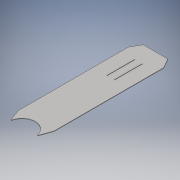
# Autodesk Inventor part: Table
Saved by Autodesk Inventor 2016 (Build 200138000, 138)
## iProperties
Created: 2015-04-25
Part Number: Table
Material: Glass
Document SubType Name: Modeling
Designer: Atok
Density: 2.18 g/cm^3
Appearance: Clear
Mass: 3769.34 g
Surface Area: 7113.49 cm^2
Volume: 1729.05 cm^3
Author: Atok
Autodesk Inventor part; units mm, degrees
ref_plane "YZ Plane" through (0, 0, 0) normal (1, 0, 0) x (0, 1, 0)
ref_plane "XZ Plane" through (0, 0, 0) normal (0, 1, 0) x (-1, 0, 0)
ref_plane "XY Plane" through (0, 0, 0) normal (0, 0, 1) x (1, 0, 0)
derived "Blade.ipt"
sketch "Sketch2" plane through (0, 0, 0) normal (0, 1, 0) x (-1, 0, 0)
  line L0 (-109.7121, -152.4) -> (109.7121, -152.4)
  line L1 (158.75, -67.4638) -> (158.75, 914.8724)
  line L2 (-158.75, 914.8724) -> (-158.75, -67.4638)
  arc A0 (-115.2875, 1017.1384) -> (115.2875, 1017.1384) centre (0, 1041.8724) ccw
  line L3 (121.3754, 1017.5583) -> (158.75, 914.8724)
  line L4 (158.75, -67.4638) -> (109.7121, -152.4)
  line L5 (-121.3754, 1017.5583) -> (-158.75, 914.8724)
  line L6 (158.75, 914.8724) -> (-158.75, 914.8724) construction
  arc A1 (121.3754, 1017.5583) -> (115.2875, 1017.1384) centre (118.3919, 1016.4724) ccw
  arc A2 (-115.2875, 1017.1384) -> (-121.3754, 1017.5583) centre (-118.3919, 1016.4724) ccw
  line L7 (-158.75, -67.4638) -> (-109.7121, -152.4)
  line L8 (0, 256.5042) -> (0, -256.5042) construction
  point P0 (0, 0)
  point P1 (0, 0)
  dimension "d9" = 160
  dimension "d10" = 150
  dimension "d11" = 3.175
  dimension "d13" = 158.75
  dimension "d14" = 152.4
  dimension "d31" = 127
  dimension "d32" = 101.6
  constraints: 18 end point, 6 point on circle, 4 tangent, 3 centre point, 2 perpendicular, 1 coincident, 1 equal radius, 1 horizontal, 1 midpoint, 1 parallel, 1 point on line, 1 symmetric about line, 1 vertical, 2 other
  measures "d9" angle of L1 L3
  measures "d10" angle of L1 L4
  measures "d11" radius of A1
  measures "d13" distance from line of point (0, 0) L1
  measures "d14" distance from line of point (0, 0) L0
  measures "d31" vertical distance of L2.start A0.centre
  measures "d32" distance from line of L6 A2.centre
extrude "Extrusion2" add sketch "Sketch2" along normal blind 5
sketch "Sketch5" plane through (0, 5, 0) normal (0, 1, 0) x (1, 0, 0)
  arc A0 (-121.3754, -1017.5583) -> (-115.2875, -1017.1384) centre (-118.3919, -1016.4724) ccw projected
  arc A1 (115.2875, -1017.1384) -> (-115.2875, -1017.1384) centre (0, -1041.8724) ccw projected
  arc A2 (115.2875, -1017.1384) -> (121.3754, -1017.5583) centre (118.3919, -1016.4724) ccw projected
  line L0 (121.3754, -1017.5583) -> (158.75, -914.8724) projected
  line L1 (158.75, -914.8724) -> (158.75, 67.4638) projected
  line L2 (158.75, 67.4638) -> (109.7121, 152.4) projected
  line L3 (109.7121, 152.4) -> (-109.7121, 152.4) projected
  line L4 (-109.7121, 152.4) -> (-158.75, 67.4638) projected
  line L5 (-158.75, 67.4638) -> (-158.75, -914.8724) projected
  line L6 (-158.75, -914.8724) -> (-121.3754, -1017.5583) projected
  line L7 (0, 146.8473) -> (0, -597.6343) construction
  line L8 (104.2991, 0) -> (-107.9294, 0) construction
  line L9 (-31.75, 0) -> (-34.798, 0)
  line L10 (-34.798, 0) -> (-34.798, -249.4096)
  line L11 (-34.798, -249.4096) -> (-31.75, -249.4096)
  line L12 (-31.75, -249.4096) -> (-31.75, 0)
  line L13 (31.75, 0) -> (34.798, 0) construction
  line L14 (34.798, 0) -> (34.798, -249.4096)
  line L15 (34.798, -249.4096) -> (31.75, -249.4096)
  line L16 (31.75, -249.4096) -> (31.75, 0)
  line L17 (34.798, 0) -> (31.75, 0)
  point P0 (0, 0)
  dimension "d27" = 249.4096
  dimension "d28" = 63.5
  dimension "d29" = 3.048
  dimension "d30" = 3.048
  constraints: 22 end point, 5 point on line, 4 parallel, 3 horizontal, 2 perpendicular, 1 collinear, 1 vertical, 1 other
  measures "d27" distance between parallel lines of L8 L11
  measures "d28" distance between parallel lines of L16 L12
  measures "d29" distance between parallel lines of L12 L10
  measures "d30" distance between parallel lines of L16 L14
extrude "Extrusion3" cut sketch "Sketch5" against normal blind 25.4 contours L12 L11 L10 L9 | L14 L15 L16 L17
equation "\"d29\" = TableCutWidth"
equation "\"d30\" = TableCutWidth"
equation "\"frgf\" = 261.49486"
equation "\"TableCutWidth\" = 3.048"
body "Solid2"
